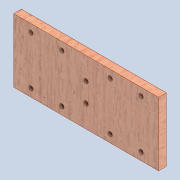
# Autodesk Inventor part: 0005-10-012
Saved by Autodesk Inventor 2020 (Build 240168000, 168)
## iProperties
Created: 2020-12-18
Part Number: 0005-10-012
Material: Wood (Maple)
Document SubType Name: Modeling
Designer: Iulian Bors
Density: 0.67 g/cm^3
Appearance: White Oak - Natural Medium Gloss
Mass: 52.2115 g
Surface Area: 240.689 cm^2
Volume: 77.9277 cm^3
Author: Iulian Bors
Subject: 012
Autodesk Inventor part; units mm, degrees
ref_plane "YZ Plane" through (0, 0, 0) normal (1, 0, 0) x (0, 1, 0)
ref_plane "XZ Plane" through (0, 0, 0) normal (0, 1, 0) x (-1, 0, 0)
ref_plane "XY Plane" through (0, 0, 0) normal (0, 0, 1) x (1, 0, 0)
sketch "Sketch1" plane through (0, 0, 0) normal (0, 0, 1) x (1, 0, 0)
  line L0 (-75, 33) -> (75, 33)
  line L1 (75, 33) -> (75, -33)
  line L2 (75, -33) -> (-75, -33)
  line L3 (-75, -33) -> (-75, 33)
  point P0 (0, 0)
  point P1 (0, 33)
  point P2 (-75, 0)
  dimension "d0" = 150
  dimension "d1" = 66
  constraints: 8 end point, 2 midpoint, 2 parallel, 1 horizontal, 1 horizontal alignment, 1 perpendicular, 1 vertical alignment
  measures "d0" distance of L0.start L0.end
  measures "d1" distance of L2.end L0.start
extrude "Extrusion1" add sketch "Sketch1" along normal blind 8
sketch "Sketch4" plane through (0, 0, 8) normal (0, 0, 1) x (1, 0, 0)
  circle A0 centre (-57, -25) radius 2.25
  circle A1 centre (-57, 25) radius 2.25
  line L0 (-75, 33) -> (-75, -33) projected
  line L1 (-75, -33) -> (75, -33) projected
  line L2 (75, 33) -> (-75, 33) projected
  circle A2 centre (-57, 0) radius 2.25
  circle A3 centre (-25, -25) radius 2.25
  circle A4 centre (-25, 0) radius 2.25
  circle A5 centre (-25, 25) radius 2.25
  circle A6 centre (57, -25) radius 2.25
  line L3 (75, -33) -> (75, 33) projected
  circle A7 centre (57, 0) radius 2.25
  circle A8 centre (57, 25) radius 2.25
  circle A9 centre (25, -25) radius 2.25
  circle A10 centre (25, 0) radius 2.25
  circle A11 centre (25, 25) radius 2.25
  circle A12 centre (0, -25) radius 2.25
  circle A13 centre (0, 25) radius 2.25
  circle A14 centre (0, 10) radius 2.25
  circle A15 centre (0, -10) radius 2.25
  point P0 (-75, 0)
  point P1 (-75, 0)
  point P2 (0, -33)
  dimension "d19" = 4.5
  dimension "d20" = 18
  dimension "d21" = 8
  dimension "d22" = 8
  dimension "d23" = 32
  dimension "d24" = 18
  dimension "d26" = 32
  dimension "d29" = 10
  dimension "d30" = 10
  constraints: 16 centre point, 15 equal radius, 13 horizontal alignment, 12 vertical alignment, 3 midpoint, 1 coincident
  measures "d19" diameter of A0
  measures "d20" distance from line of A0.centre L0
  measures "d21" distance from line of A0.centre L1
  measures "d22" distance from line of L2 A1.centre
  measures "d23" distance of A3.centre A0.centre
  measures "d24" distance from line of L3 A6.centre
  measures "d26" distance of A6.centre A9.centre
  measures "d29" vertical distance of A14.centre A10.centre
  measures "d30" vertical distance of A10.centre A15.centre
extrude "Extrusion4" cut sketch "Sketch4" against normal through all contours A0 | A1 | A3 | A5 | A6 | A8 | A9 | A11 | A14 | A15
equation "\"d22\" = d21"
equation "\"d24\" = d20"
equation "\"d26\" = d23"
body "Solid1"
